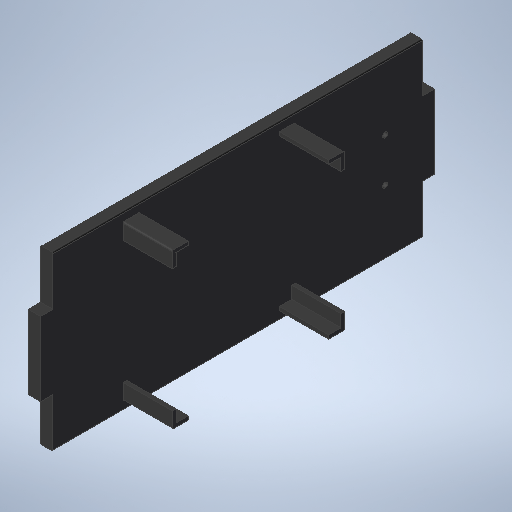
# Autodesk Inventor part: Chassis_Upper_Portion
Saved by Autodesk Inventor 2025 (Build 290162000, 162)
## iProperties
Created: 2024-06-26
Part Number: Chassis_Upper_Portion
Material: Generic
Document SubType Name: Modeling
Designer: sml6042
Density: 1 g/cm^3
Appearance: Default
Author: sml6042
Autodesk Inventor part; units mm, degrees
ref_plane "YZ Plane" through (0, 0, 0) normal (1, 0, 0) x (0, 1, 0)
ref_plane "XZ Plane" through (0, 0, 0) normal (0, 1, 0) x (-1, 0, 0)
ref_plane "XY Plane" through (0, 0, 0) normal (0, 0, 1) x (1, 0, 0)
sketch "Sketch1" plane through (0, 0, 0) normal (1, 0, 0) x (0, 1, 0)
  line L0 (0, 0) -> (70, 0)
  line L1 (70, 0) -> (70, -150)
  line L2 (70, -150) -> (0, -150)
  line L3 (0, -150) -> (0, 0)
  dimension "d0" = 70
  dimension "d1" = 150
  constraints: 8 end point, 2 parallel, 1 horizontal, 1 perpendicular
  measures "d0" distance of L1.end L2.end
  measures "d1" distance of L0.end L1.end
extrude "Extrusion1" add sketch "Sketch1" along normal blind 5
sketch "Sketch2" plane through (0, 0, 0) normal (0, 0, 1) x (1, 0, 0)
  line L0 (0, 0) -> (0, 20)
  line L1 (0, 0) -> (0, 70) projected
  line L2 (0, 20) -> (0, 20)
  line L3 (0, 20) -> (0, 50)
  line L4 (0, 50) -> (5, 50)
  line L5 (5, 50) -> (5, 20)
  line L6 (5, 20) -> (0, 20)
  dimension "d4" = 20
  dimension "d5" = 0
  dimension "d6" = 30
  dimension "d7" = 5
  constraints: 12 end point, 4 perpendicular, 2 point on line, 1 horizontal
  measures "d4" distance of L0.start L0.end
  measures "d5" distance of L0.end L2.end
  measures "d6" distance of L2.end L3.end
  measures "d7" distance of L3.end L4.end
extrude "Extrusion2" add sketch "Sketch2" along normal blind 5
sketch "Sketch3" plane through (0, 0, -150) normal (0, 0, -1) x (-1, 0, 0)
  line L0 (0, 0) -> (0, 0)
  line L1 (0, 0) -> (-5, 0) projected
  line L2 (0, 0) -> (0, 20)
  line L3 (0, 20) -> (-5, 20)
  line L4 (-5, 20) -> (-5, 50)
  line L5 (-5, 50) -> (0, 50)
  line L6 (0, 50) -> (0, 20)
  dimension "d10" = 0
  dimension "d11" = 20
  dimension "d12" = 5
  dimension "d13" = 30
  constraints: 12 end point, 4 perpendicular, 2 point on line, 1 collinear
  measures "d10" distance of L0.start L0.end
  measures "d11" distance of L0.end L2.end
  measures "d12" distance of L2.end L3.end
  measures "d13" distance of L3.end L4.end
extrude "Extrusion3" add sketch "Sketch3" along normal blind 5
sketch "Sketch4" plane through (5, 0, 0) normal (1, 0, 0) x (0, 0, -1)
  line L0 (0, 0) -> (150, 0) projected
  line L1 (0, 0) -> (0, 5)
  line L2 (0, 70) -> (0, 0) projected
  line L3 (0, 5) -> (28.5, 5)
  line L4 (30, 5) -> (30, 65)
  line L5 (30, 65) -> (97, 65)
  line L6 (97, 65) -> (97, 5)
  line L7 (97, 5) -> (30, 5)
  line L8 (30, 65) -> (28.5, 65)
  line L9 (28.5, 65) -> (28.5, 60)
  line L10 (28.5, 60) -> (30, 60)
  line L11 (28.5, 65) -> (28.5, 66.5)
  line L12 (28.5, 66.5) -> (35, 66.5)
  line L13 (35, 66.5) -> (35, 65)
  line L14 (28.5, 5) -> (28.5, 10)
  line L15 (28.5, 10) -> (30, 10)
  line L16 (28.5, 5) -> (28.5, 3.5)
  line L17 (28.5, 3.5) -> (35, 3.5)
  line L18 (35, 3.5) -> (35, 5)
  line L19 (97, 5) -> (98.5, 5)
  line L20 (98.5, 5) -> (98.5, 10)
  line L21 (98.5, 10) -> (97, 10)
  line L22 (98.5, 5) -> (98.5, 3.5)
  line L23 (98.5, 3.5) -> (92, 3.5)
  line L24 (92, 3.5) -> (92, 5)
  line L25 (92, 65) -> (92, 66.5)
  line L26 (92, 66.5) -> (98.5, 66.5)
  line L27 (98.5, 66.5) -> (98.5, 60)
  line L28 (98.5, 60) -> (97, 60)
  dimension "d16" = 5
  dimension "d17" = 30
  dimension "d18" = 60
  dimension "d19" = 67
  dimension "d20" = 1.5
  dimension "d21" = 5
  dimension "d22" = 1.5
  dimension "d23" = 6.5
  dimension "d24" = 5
  dimension "d25" = 1.5
  dimension "d26" = 1.5
  dimension "d27" = 5
  dimension "d28" = 1.5
  dimension "d29" = 6.5
  dimension "d30" = 6.5
  dimension "d31" = 6.5
  constraints: 54 end point, 27 point on line, 11 perpendicular, 2 horizontal
  measures "d16" distance of L0.start L1.end
  measures "d17" distance of L1.end L4.start
  measures "d18" distance of L4.start L4.end
  measures "d19" distance of L4.end L5.end
  measures "d20" distance of L4.end L8.end
  measures "d21" distance of L8.end L9.end
  measures "d22" distance of L8.end L11.end
  measures "d23" distance of L11.end L12.end
  measures "d24" distance of L3.end L14.end
  measures "d25" distance of L3.end L16.end
  measures "d26" distance of L6.end L19.end
  measures "d27" distance of L19.end L20.end
  measures "d28" distance of L19.end L22.end
  measures "d29" distance of L22.end L23.end
  measures "d30" distance of L25.end L26.end
  measures "d31" distance of L26.end L27.end
extrude "Extrusion4" add sketch "Sketch4" along normal blind 20 contours L7 L18 L17 L16 L14 L15 L4 | L10 L9 L8 L4 | L7 L19 L22 L23 L24 | L8 L11 L12 L13 L5 | L6 L21 L20 L19 | L25 L26 L27 L28 L6 L5
fillet "Fillet1" radius 0.5 8 edges at (5, 70, -75) (0, 70, -75) (5, 0, -75) (0, 0, -75) (15, 3.5, -28.5) (15, 66.5, -28.5) (15, 66.5, -98.5) (15, 3.5, -98.5)
sketch "Sketch5" plane through (0, 0, 0) normal (-1, 0, 0) x (0, 0, 1)
  line L0 (-155, 20) -> (-155, 50) projected
  line L1 (-155, 35) -> (-135, 35)
  line L2 (-135, 35) -> (-135, 43.825)
  line L3 (-135, 43.825) -> (-135, 26.175)
  circle A0 centre (-135, 43.825) radius 1.025
  circle A1 centre (-135, 26.175) radius 1.025
  point P0 (0, 0)
  dimension "d35" = 20
  dimension "d36" = 8.825
  dimension "d37" = 17.65
  dimension "d38" = 2.05
  dimension "d39" = 2.05
  constraints: 6 end point, 2 centre point, 2 coincident, 1 horizontal, 1 midpoint, 1 perpendicular, 1 point on line
  measures "d35" distance of L1.start L1.end
  measures "d36" distance of L1.end L2.end
  measures "d37" distance of L2.end L3.end
  measures "d38" diameter of A0
  measures "d39" diameter of A1
extrude "Extrusion5" cut sketch "Sketch5" against normal through all
body "Solid1"
